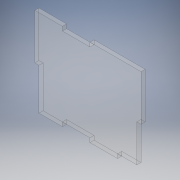
# Autodesk Inventor part: front_left
Saved by Autodesk Inventor 2017.2 (Build 212233000, 233)
## iProperties
Created: 2017-06-02
Part Number: front_left
Material: Generic
Document SubType Name: Modeling
Designer: SandeepSH
Density: 1 g/cm^3
Appearance: Polycarbonate - Clear
Author: SandeepSH
Autodesk Inventor part; units mm, degrees
ref_plane "YZ Plane" through (0, 0, 0) normal (1, 0, 0) x (0, 1, 0)
ref_plane "XZ Plane" through (0, 0, 0) normal (0, 1, 0) x (-1, 0, 0)
ref_plane "XY Plane" through (0, 0, 0) normal (0, 0, 1) x (1, 0, 0)
sketch "Sketch1" plane through (0, 0, 0) normal (0, 0, 1) x (1, 0, 0)
  line L0 (-38.5, -31.5) -> (38.5, -31.5)
  line L1 (38.5, -31.5) -> (38.5, 31.5)
  line L2 (38.5, 31.5) -> (-38.5, 31.5)
  line L3 (-38.5, 31.5) -> (-38.5, -31.5)
  line L4 (-38.5, -31.5) -> (38.5, 31.5) construction
  line L5 (38.5, -31.5) -> (-38.5, 31.5) construction
  point P0 (0, 0)
  dimension "d0" = 77
  dimension "d1" = 63
  constraints: 12 end point, 2 midpoint, 2 parallel, 1 horizontal, 1 perpendicular
  measures "d0" distance of L2.end L1.end
  measures "d1" distance of L1.end L0.end
extrude "Extrusion1" add sketch "Sketch1" along normal blind 3
sketch "Sketch2" plane through (0, 0, 3) normal (0, 0, 1) x (1, 0, 0)
  line L0 (-38.5, 31.5) -> (-38.5, -31.5) projected
  line L1 (-38.5, -31.5) -> (-35.5, -31.5)
  line L2 (-35.5, -31.5) -> (-35.5, -1.5)
  line L3 (-35.5, -1.5) -> (-38.5, -1.5)
  line L4 (-38.5, -1.5) -> (-38.5, -31.5)
  line L5 (-38.5, -31.5) -> (38.5, -31.5) projected
  line L6 (38.5, -31.5) -> (35.5, -31.5)
  line L7 (35.5, -31.5) -> (35.5, -1.5)
  line L8 (35.5, -1.5) -> (38.5, -1.5)
  line L9 (38.5, -1.5) -> (38.5, -31.5)
  line L10 (-18.5, -31.5) -> (1.5, -31.5)
  line L11 (1.5, -31.5) -> (1.5, -28.5)
  line L12 (1.5, -28.5) -> (-18.5, -28.5)
  line L13 (-18.5, -28.5) -> (-18.5, -31.5)
  line L14 (35.5, -31.5) -> (21.5, -31.5)
  line L15 (21.5, -31.5) -> (21.5, -28.5)
  line L16 (21.5, -28.5) -> (35.5, -28.5)
  line L17 (35.5, -28.5) -> (35.5, -31.5)
  point P0 (0, 0)
  dimension "d4" = 3
  dimension "d5" = 30
  dimension "d6" = 3
  dimension "d7" = 30
  dimension "d8" = 20
  dimension "d9" = 3
  dimension "d10" = 20
  dimension "d11" = 3
  dimension "d12" = 20
  constraints: 32 end point, 8 parallel, 4 horizontal, 4 perpendicular, 1 point on line
  measures "d4" distance of L3.end L2.end
  measures "d5" distance of L2.end L1.end
  measures "d6" distance of L7.end L8.end
  measures "d7" distance of L6.end L7.end
  measures "d8" distance of L12.end L11.end
  measures "d9" distance of L11.end L10.end
  measures "d10" distance between parallel lines of L4 L13
  measures "d11" distance of L14.end L15.end
  measures "d12" distance between parallel lines of L15 L11
extrude "Extrusion2" cut sketch "Sketch2" against normal through all
sketch "Sketch3" plane through (0, 0, 3) normal (0, 0, 1) x (1, 0, 0)
  line L0 (38.5, 31.5) -> (-38.5, 31.5) projected
  line L1 (-18.5, 31.5) -> (1.5, 31.5)
  line L2 (1.5, 31.5) -> (1.5, 28.5)
  line L3 (1.5, 28.5) -> (-18.5, 28.5)
  line L4 (-18.5, 28.5) -> (-18.5, 31.5)
  line L5 (-38.5, 31.5) -> (-38.5, -1.5) projected
  point P0 (0, 0)
  dimension "d15" = 20
  dimension "d16" = 3
  dimension "d17" = 20
  constraints: 8 end point, 2 parallel, 1 horizontal, 1 perpendicular, 1 point on line
  measures "d15" distance of L2.end L3.end
  measures "d16" distance of L1.end L2.end
  measures "d17" distance between parallel lines of L4 L5
extrude "Extrusion3" cut sketch "Sketch3" against normal blind 3
body "Solid1"
